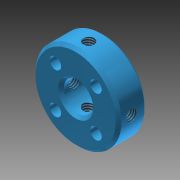
# Autodesk Inventor part: None_Magnet_Extender_Split_Bottom
Saved by Autodesk Inventor 2015 (Build 190159000, 159)
## iProperties
Created: 2015-01-06
Part Number: None_Magnet_Extender_Split_Bottom
Material: Aluminum 6061
Document SubType Name: Modeling
Designer: ice
Mass: 1.54881 g
Surface Area: 8.35285 cm^2
Volume: 0.573632 cm^3
Density: 2.7 g/cm^3
Appearance: Aluminum - Flat
Author: ice
Autodesk Inventor part; units mm, degrees
sketch "Sketch1" plane through (0, 0, 0) normal (1, 0, 0) x (0, 1, 0)
  line L0 (15.4, 5) -> (15.4, 2.55)
  line L1 (15.4, 2.55) -> (20.4, 2.55)
  line L2 (20.8521, 0) -> (14.3565, 0)
  line L3 (15.4, 5) -> (15.4, 7.5)
  line L4 (15.4, 7.5) -> (20.4, 7.5)
  line L5 (20.4, 7.5) -> (20.4, 2.55)
  line L6 (20.4, 5.025) -> (20.4, 2.55)
  line L7 (20.4, 7.5) -> (20.4, 7)
  line L8 (20.4, 7.5) -> (19.9, 7.5)
  line L9 (20.4, 2.55) -> (20.4, 3.05)
  line L10 (20.4, 2.55) -> (19.9, 2.55)
  line L11 (15.4, 2.55) -> (15.9, 2.55)
  line L12 (15.4, 2.55) -> (15.4, 3.05)
  line L13 (15.4, 7.5) -> (15.9, 7.5)
  line L14 (15.4, 7.5) -> (15.4, 7)
  point P0 (0, 0)
  dimension "d218" = 5
  dimension "d264" = 5
  dimension "d265" = 4.95
  dimension "d266" = 2.55
  dimension "d267" = 5.025
  dimension "d306" = 7.5
  dimension "d339" = 0.5
  dimension "d340" = 0.5
  dimension "d341" = 0.5
  dimension "d342" = 0.5
  dimension "d343" = 0.5
  dimension "d344" = 0.5
  dimension "d345" = 0.5
  dimension "d346" = 0.5
  constraints: 30 end point, 8 point on line, 2 perpendicular, 2 vertical, 1 collinear, 1 horizontal, 1 midpoint
  measures "d218" distance of L0.end L1.end
  measures "d264" distance of L3.end L4.end
  measures "d265" distance of L3.end L0.end
  measures "d266" distance from line of L2 L0.end
  measures "d267" distance from line of L2 L6.start
  measures "d306" vertical distance of L2.start L4.end
  measures "d339" distance of L4.end L7.end
  measures "d340" distance of L4.end L8.end
  measures "d341" distance of L1.end L9.end
  measures "d342" distance of L1.end L10.end
  measures "d343" distance of L0.end L11.end
  measures "d344" distance of L0.end L12.end
  measures "d345" distance of L3.end L13.end
  measures "d346" distance of L3.end L14.end
revolve "Revolution1" add sketch "Sketch1" angle 360 about axis through (0, 20.8521, 0) along (0, -1, 0)
ref_plane "Work Plane12" through (0, 0, 5) normal (0, 0, 1) x (1, 0, 0)
ref_plane "Work Plane3" through (5, 0, 0) normal (1, 0, 0) x (0, 1, 0)
sketch "Sketch10" plane through (0, 20.4, 0) normal (0, 1, 0) x (1, 0, 0)
  line L0 (0, 0) -> (2.55, 0)
  circle A0 centre (0, 0) radius 2.55 projected
  line L1 (2.55, 0) -> (7.5, 0)
  circle A1 centre (0, 0) radius 7.5 projected
  line L2 (0, 0) -> (3.5355, -3.5355)
  line L3 (0, 0) -> (5, 0) construction
  line L4 (0, 0) -> (3.5355, 3.5355)
  line L5 (0, 0) -> (-3.5355, 3.5355)
  line L6 (0, 0) -> (5, 0) construction
  line L7 (0, 0) -> (-3.5355, -3.5355)
  line L8 (0, 0) -> (5, 0) construction
  circle A2 centre (3.5355, 3.5355) radius 1
  circle A3 centre (-3.5355, 3.5355) radius 1
  circle A4 centre (-3.5355, -3.5355) radius 1
  circle A5 centre (3.5355, -3.5355) radius 1
  dimension "d268" = 4.95
  dimension "d269" = 2.55
  dimension "d270" = 5
  dimension "d271" = 45
  dimension "d272" = 5
  dimension "d273" = 5
  dimension "d274" = 135
  dimension "d275" = 5
  dimension "d276" = 135
  dimension "d335" = 2
  dimension "d336" = 2
  dimension "d337" = 2
  dimension "d338" = 2
  constraints: 18 end point, 4 centre point, 4 horizontal, 3 coincident, 3 equal length, 2 horizontal alignment, 1 perpendicular, 1 point on line, 2 other
  measures "d268" distance of L0.end L1.end
  measures "d269" distance of L0.end L0.start
  measures "d270" distance of L2.start L2.end
  measures "d271" angle of L2 L3
  measures "d272" distance of L2.start L4.end
  measures "d273" distance of L2.start L5.end
  measures "d274" angle of L6 L5
  measures "d275" distance of L2.start L7.end
  measures "d276" angle of L7 L8
  measures "d335" diameter of A2
  measures "d336" diameter of A3
  measures "d337" diameter of A4
  measures "d338" diameter of A5
hole "Hole6" at (3.5355, 20.4, -3.5355) at (3.5355, 20.4, 3.5355) at (-3.5355, 20.4, 3.5355) at (-3.5355, 20.4, -3.5355) direction (0, -1, 0) diameter 2 end through all counterbore diameter 4.1 counterbore depth 1.8
ref_plane "Work Plane15" through (0, 0, 7.5) normal (0, 0, 1) x (1, 0, 0)
sketch "Sketch12" plane through (0, 0, 7.5) normal (0, 0, 1) x (1, 0, 0)
  point P0 (0, 17.65)
hole "Hole7" at (0, 17.65, 7.5) direction (0, 0, -1) diameter 1.9 end through all
ref_plane "Work Plane8" through (7.5, 0, 0) normal (1, 0, 0) x (0, 1, 0)
sketch "Sketch13" plane through (7.5, 0, 0) normal (1, 0, 0) x (0, 1, 0)
  line L0 (20.4, 7.5) -> (20.4, -7.5) projected
  line L1 (20.4, 0) -> (15.4, 0)
  line L2 (15.4, 7.5) -> (15.4, -7.5) projected
  line L3 (15.4, 0) -> (17.65, 0)
  point P0 (0, 0)
  dimension "d295" = 2.25
  constraints: 4 end point, 2 midpoint, 1 point on line
  measures "d295" distance of L1.end L3.end
hole "Hole8" at (7.5, 17.65, 0) direction (-1, 0, 0) diameter 1.9 end through all
chamfer "Chamfer5" distance 0.5 angle 45 4 edges at (0, 20.4, -7.5) (0, 15.4, -7.5) (0, 20.4, -2.55) (0, 15.4, -2.55)
ref_plane "Work Plane14" through (0, 15.4, 0) normal (0, -1, 0) x (1, 0, 0)
ref_plane "Work Plane16" through (-3.5355, 18.6, -3.5355) normal (0, 1, 0) x (1, 0, 0)
ref_plane "Work Plane17" through (3.5355, 18.6, -3.5355) normal (0, 1, 0) x (1, 0, 0)
ref_plane "Work Plane18" through (-3.5355, 18.6, 3.5355) normal (0, 1, 0) x (1, 0, 0)
ref_plane "Work Plane19" through (3.5355, 18.6, 3.5355) normal (0, 1, 0) x (1, 0, 0)
thread "Thread13" size "M2x0.4" class "6H" standard "ANSI Metric M Profile" full length
thread "Thread15" size "M2x0.4" class "6H" standard "ANSI Metric M Profile" full length
thread "Thread17" size "M2x0.4" class "6H" standard "ANSI Metric M Profile" full length
thread "Thread18" size "M2x0.4" class "6H" standard "ANSI Metric M Profile" full length
ref_plane "Work Plane20" through (0, 0, 2.5) normal (0, 0, 1) x (1, 0, 0)
ref_plane "Work Plane22" through (2.5, 0, 0) normal (1, 0, 0) x (0, 1, 0)
body "Solid1"
